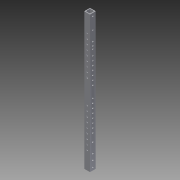
# Autodesk Inventor part: Chassis Part4 (26x28)
Saved by Autodesk Inventor 2013 (Build 170138000, 138)
## iProperties
Created: 2013-01-05
Part Number: Chassis Part4 (26x28)
Material: Aluminum 6061
Document SubType Name: Modeling
Designer: Moses
Density: 2.71 g/cm^3
Mass: 441.537 g
Surface Area: 1087.3 cm^2
Volume: 162.929 cm^3
Author: Moses
Autodesk Inventor part; units mm, degrees
ref_plane "YZ Plane" through (0, 0, 0) normal (1, 0, 0) x (0, 1, 0)
ref_plane "XZ Plane" through (0, 0, 0) normal (0, 1, 0) x (-1, 0, 0)
ref_plane "XY Plane" through (0, 0, 0) normal (0, 0, 1) x (1, 0, 0)
sketch "Sketch1" plane through (0, 0, 0) normal (0, 1, 0) x (-1, 0, 0)
  line L0 (0, 25.4) -> (25.4, 25.4)
  line L1 (25.4, 25.4) -> (25.4, 0)
  line L2 (25.4, 0) -> (0, 0)
  line L3 (0, 0) -> (0, 25.4)
  line L4 (22.225, 22.225) -> (3.175, 22.225)
  line L5 (3.175, 22.225) -> (3.175, 3.175)
  line L6 (3.175, 3.175) -> (22.225, 3.175)
  line L7 (22.225, 3.175) -> (22.225, 22.225)
  dimension "d0" = 25.4
  dimension "d1" = 25.4
  dimension "d2" = 3.175
  constraints: 16 end point, 4 parallel, 2 perpendicular, 1 coincident, 1 horizontal, 3 other
  measures "d0" distance of L1.end L2.end
  measures "d1" distance of L0.end L1.end
  measures "d2" distance between parallel lines of L0 L4
extrude "Extrusion1" add sketch "Sketch1" along normal blind 609.6
sketch "Sketch2" plane through (-25.4, 0, 25.4) normal (0, 0, 1) x (1, 0, 0)
  line L0 (25.4, 0) -> (0, 0) projected
  line L1 (0, 609.6) -> (25.4, 609.6) projected
  line L2 (12.7, 609.6) -> (12.7, 0) construction
  line L3 (12.7, 0) -> (12.7, 13.97) construction
  circle A0 centre (12.7, 13.97) radius 3.302
  circle A1 centre (12.7, 35.513) radius 3.302
  circle A2 centre (12.7, 57.0559) radius 3.302
  circle A3 centre (12.7, 78.5989) radius 3.302
  circle A4 centre (12.7, 100.1419) radius 3.302
  circle A5 centre (12.7, 121.6848) radius 3.302
  circle A6 centre (12.7, 143.2278) radius 3.302
  circle A7 centre (12.7, 164.7707) radius 3.302
  circle A8 centre (12.7, 186.3137) radius 3.302
  circle A9 centre (12.7, 207.8567) radius 3.302
  circle A10 centre (12.7, 229.3996) radius 3.302
  circle A11 centre (12.7, 250.9426) radius 3.302
  circle A12 centre (12.7, 272.4856) radius 3.302
  circle A13 centre (12.7, 294.0285) radius 3.302
  circle A14 centre (12.7, 315.5715) radius 3.302
  circle A15 centre (12.7, 337.1144) radius 3.302
  circle A16 centre (12.7, 358.6574) radius 3.302
  circle A17 centre (12.7, 380.2004) radius 3.302
  circle A18 centre (12.7, 401.7433) radius 3.302
  circle A19 centre (12.7, 423.2863) radius 3.302
  circle A20 centre (12.7, 444.8293) radius 3.302
  circle A21 centre (12.7, 466.3722) radius 3.302
  circle A22 centre (12.7, 487.9152) radius 3.302
  circle A23 centre (12.7, 509.4581) radius 3.302
  circle A24 centre (12.7, 531.0011) radius 3.302
  circle A25 centre (12.7, 552.5441) radius 3.302
  circle A26 centre (12.7, 574.087) radius 3.302
  circle A27 centre (12.7, 595.63) radius 3.302
  dimension "d5" = 13.97
  dimension "d6" = 6.604
  dimension "d7" = 609.6
  dimension "d10" = 21.543
  constraints: 28 centre point, 4 end point, 2 midpoint, 1 coincident, 1 point on line, 1 vertical, 54 other
  measures "d5" distance of L2.end L3.end
  measures "d6" diameter of A0
  measures "d7" distance of L0.end L1.start
  measures "d10" distance of A0.centre A1.centre
extrude "Extrusion2" cut sketch "Sketch2" against normal through all contours A3 | A4 | A5 | A6 | A7 | A8 | A9 | A10 | A11 | A16 | A17 | A18 | A19 | A20 | A21 | A22 | A23 | A24
sketch "Sketch3" plane through (-25.4, 0, 0) normal (-1, 0, 0) x (0, 0, 1)
  line L0 (25.4, 0) -> (25.4, 609.6) projected
  line L1 (0, 0) -> (0, 609.6) projected
  line L2 (0, 229.3996) -> (25.4, 229.3996) construction
  line L3 (12.7, 543.7011) -> (12.7, 499.2511) construction
  line L4 (12.7, 405.6004) -> (12.7, 354.8004) construction
  line L5 (12.7, 251.6246) -> (12.7, 207.1746) construction
  line L6 (12.7, 110.3489) -> (12.7, 65.8989) construction
  circle A0 centre (12.7, 543.7011) radius 3.302
  circle A1 centre (12.7, 499.2511) radius 3.302
  circle A2 centre (12.7, 405.6004) radius 3.302
  circle A3 centre (12.7, 354.8004) radius 3.302
  circle A4 centre (12.7, 251.6246) radius 3.302
  circle A5 centre (12.7, 207.1746) radius 3.302 construction
  circle A6 centre (12.7, 110.3489) radius 3.302
  circle A7 centre (12.7, 65.8989) radius 3.302
  line L7 (0, 304.8) -> (25.4, 304.8) construction
  line L8 (12.7, 330.2) -> (12.7, 279.4) construction
  circle A8 centre (12.7, 330.2) radius 3.302
  circle A9 centre (12.7, 279.4) radius 3.302
  line L9 (25.4, 0) -> (0, 0) projected
  line L10 (0, 609.6) -> (25.4, 609.6) projected
  circle A10 centre (12.7, 596.9) radius 3.302
  line L11 (12.7, 596.9) -> (12.7, 609.6) construction
  line L12 (12.7, 0) -> (12.7, 12.7) construction
  circle A11 centre (12.7, 12.7) radius 3.302
  line L13 (0, 88.1239) -> (25.4, 88.1239) construction
  line L14 (0, 521.4761) -> (25.4, 521.4761) construction
  line L15 (12.7, 12.7) -> (12.7, 40.4989) construction
  circle A12 centre (12.7, 40.4989) radius 3.302
  line L16 (0, 13.97) -> (25.4, 13.97) construction
  line L17 (0, 35.513) -> (25.4, 35.513) construction
  line L18 (0, 57.0559) -> (25.4, 57.0559) construction
  line L19 (0, 78.5989) -> (25.4, 78.5989) construction
  line L20 (0, 100.1419) -> (25.4, 100.1419) construction
  line L21 (0, 121.6848) -> (25.4, 121.6848) construction
  line L22 (0, 143.2278) -> (25.4, 143.2278) construction
  line L23 (0, 164.7707) -> (25.4, 164.7707) construction
  line L24 (0, 186.3137) -> (25.4, 186.3137) construction
  line L25 (0, 207.8567) -> (25.4, 207.8567) construction
  line L26 (0, 229.3996) -> (25.4, 229.3996) construction
  line L27 (0, 250.9426) -> (25.4, 250.9426) construction
  line L28 (0, 272.4856) -> (25.4, 272.4856) construction
  line L29 (0, 294.0285) -> (25.4, 294.0285) construction
  line L30 (0, 315.5715) -> (25.4, 315.5715) construction
  line L31 (0, 337.1144) -> (25.4, 337.1144) construction
  line L32 (0, 358.6574) -> (25.4, 358.6574) construction
  line L33 (0, 380.2004) -> (25.4, 380.2004) construction
  line L34 (0, 401.7433) -> (25.4, 401.7433) construction
  line L35 (0, 423.2863) -> (25.4, 423.2863) construction
  line L36 (0, 444.8293) -> (25.4, 444.8293) construction
  line L37 (0, 466.3722) -> (25.4, 466.3722) construction
  line L38 (0, 487.9152) -> (25.4, 487.9152) construction
  line L39 (0, 509.4581) -> (25.4, 509.4581) construction
  line L40 (0, 531.0011) -> (25.4, 531.0011) construction
  line L41 (0, 552.5441) -> (25.4, 552.5441) construction
  line L42 (0, 574.087) -> (25.4, 574.087) construction
  line L43 (0, 595.63) -> (25.4, 595.63) construction
  line L44 (3.175, 534.3031) -> (3.175, 527.6991) projected
  line L45 (3.175, 383.5024) -> (3.175, 376.8984) projected
  line L46 (3.175, 81.9009) -> (3.175, 75.2969) projected
  line L47 (3.175, 232.7016) -> (3.175, 226.0976) projected
  point P0 (12.7, 304.8)
  point P1 (12.7, 88.1239)
  point P2 (12.7, 521.4761)
  point P3 (12.7, 380.2004)
  point P4 (12.7, 229.3996)
  dimension "d17" = 44.45
  dimension "d18" = 50.8
  dimension "d19" = 44.45
  dimension "d20" = 44.45
  dimension "d21" = 6.604
  dimension "d22" = 6.604
  dimension "d23" = 6.604
  dimension "d24" = 6.604
  dimension "d25" = 6.604
  dimension "d26" = 6.604
  dimension "d27" = 6.604
  dimension "d28" = 6.604
  dimension "d31" = 50.8
  dimension "d32" = 6.604
  dimension "d33" = 6.604
  dimension "d40" = 12.7
  dimension "d41" = 6.604
  dimension "d42" = 12.7
  dimension "d43" = 6.604
  dimension "d64" = 25.4
  dimension "d65" = 6.604
  dimension "d66" = 13.97
  dimension "d67" = 609.6
  dimension "d70" = 21.543
  dimension "d76" = 9.525
  dimension "d77" = 9.525
  constraints: 80 end point, 15 midpoint, 13 centre point, 12 coincident, 8 point on line, 5 collinear, 5 perpendicular, 3 vertical, 81 other
  measures "d17" distance of L3.start L3.end
  measures "d18" distance of L4.start L4.end
  measures "d19" distance of L5.start L5.end
  measures "d20" distance of L6.start L6.end
  measures "d21" diameter of A0
  measures "d22" diameter of A1
  measures "d23" diameter of A2
  measures "d24" diameter of A3
  measures "d25" diameter of A4
  measures "d26" diameter of A5
  measures "d27" diameter of A6
  measures "d28" diameter of A7
  measures "d31" distance of L8.start L8.end
  measures "d32" diameter of A8
  measures "d33" diameter of A9
  measures "d40" distance from line of L10 L11.start
  measures "d41" diameter of A10
  measures "d42" distance of L12.start L12.end
  measures "d43" diameter of A11
  measures "d64" distance of L6.end L15.end
  measures "d65" diameter of A12
  measures "d66" distance between parallel lines of L9 L16
  measures "d67" distance of L1.start L1.end
  measures "d70" distance of L16.start L17.start
  measures "d76" distance between parallel lines of L40 L14
  measures "d77" distance between parallel lines of L19 L13
extrude "Extrusion3" cut sketch "Sketch3" against normal through all contours A0 | A1 | A6 | A7 | A8 | A9 | A10 | A11 | A12
sketch "Sketch4" plane through (0, 0, 25.4) normal (1, 0, 0) x (0, 0, -1)
  circle A0 centre (12.7, 330.2) radius 3.302 construction
  circle A1 centre (12.7, 279.4) radius 3.302 construction
  line L0 (0, 0) -> (0, 609.6) projected
  line L1 (12.7, 330.2) -> (12.7, 349.25) construction
  line L2 (12.7, 279.4) -> (12.7, 260.35) construction
  circle A2 centre (12.7, 349.25) radius 3.302
  circle A3 centre (12.7, 260.35) radius 3.302
  line L3 (25.4, 0) -> (0, 0) projected
  line L4 (0, 609.6) -> (25.4, 609.6) projected
  line L5 (12.7, 609.6) -> (12.7, 0) construction
  circle A4 centre (12.7, 469.9) radius 3.302
  circle A5 centre (12.7, 482.6) radius 3.302
  circle A6 centre (12.7, 241.3) radius 3.302
  circle A7 centre (12.7, 222.25) radius 3.302
  circle A8 centre (12.7, 203.2) radius 3.302
  circle A9 centre (12.7, 184.15) radius 3.302
  circle A10 centre (12.7, 165.1) radius 3.302
  circle A11 centre (12.7, 368.3) radius 3.302
  circle A12 centre (12.7, 387.35) radius 3.302
  circle A13 centre (12.7, 406.4) radius 3.302
  circle A14 centre (12.7, 425.45) radius 3.302
  circle A15 centre (12.7, 444.5) radius 3.302
  circle A16 centre (12.7, 146.05) radius 3.302
  dimension "d46" = 19.05
  dimension "d47" = 19.05
  dimension "d48" = 6.604
  dimension "d49" = 6.604
  dimension "d52" = 6.604
  dimension "d53" = 139.7
  dimension "d85" = 12.7
  dimension "d88" = 19.05
  dimension "d95" = 19.05
  constraints: 15 centre point, 6 end point, 2 coincident, 2 midpoint, 2 point on line, 2 vertical, 1 collinear, 1 equal radius, 1 parallel, 22 other
  measures "d46" distance of L1.start L1.end
  measures "d47" distance of L2.start L2.end
  measures "d48" diameter of A2
  measures "d49" diameter of A3
  measures "d52" diameter of A4
  measures "d53" distance from line of L4 A4.centre
  measures "d85" distance of A4.centre A5.centre
  measures "d88" distance of A3.centre A6.centre
  measures "d95" distance of A2.centre A11.centre
extrude "Extrusion4" cut sketch "Sketch4" against normal blind 25.4
equation "\"d19\" = d17"
equation "\"d20\" = d17"
equation "\"d22\" = d21"
equation "\"d23\" = d21"
equation "\"d24\" = d21"
equation "\"d25\" = d21"
equation "\"d26\" = d21"
equation "\"d27\" = d21"
equation "\"d28\" = d21"
equation "\"d31\" = d18"
equation "\"d32\" = d21"
equation "\"d33\" = d21"
equation "\"d41\" = d21"
equation "\"d42\" = d40"
equation "\"d43\" = d21"
equation "\"d70\" = -0.0740741 * d66 + 0.037037 * d67"
equation "\"d76\" = d77"
body "Solid1"
